nixal_reprap4040_XtensionerHolder (Autodesk Fusion 360 design; units mm, degrees)
Autodesk Fusion 360 part; units mm, degrees
sketch "Sketch1" plane through (0, 0, 0) normal (0, 1, 0) x (1, 0, 0)
  line L0 (2, 0) -> (6.3, 0)
  line L1 (8.3, 2) -> (8.3, 22.7)
  line L2 (6.3, 24.7) -> (2, 24.7)
  line L3 (0, 22.7) -> (0, 2)
  line L4 (-2, 26.2) -> (10.3, 26.2)
  line L5 (12.3, 24.2) -> (12.3, 0.5)
  line L6 (10.3, -1.5) -> (-2, -1.5)
  line L7 (-4, 0.5) -> (-4, 24.2)
  line L8 (0, 24.7) -> (8.3, 0) construction
  line L9 (8.3, 24.7) -> (0, 0) construction
  circle A0 centre (4.15, 12.35) radius 1.65
  line L10 (7.4, 9.1) -> (0.9, 15.6) construction
  line L11 (0.9, 9.1) -> (7.4, 15.6) construction
  circle A1 centre (4.15, 12.35) radius 3.25
  arc A2 (2, 24.7) -> (0, 22.7) centre (2, 22.7) ccw
  arc A3 (8.3, 22.7) -> (6.3, 24.7) centre (6.3, 22.7) ccw
  arc A4 (0, 2) -> (2, 0) centre (2, 2) ccw
  arc A5 (6.3, 0) -> (8.3, 2) centre (6.3, 2) ccw
  arc A6 (-2, 26.2) -> (-4, 24.2) centre (-2, 24.2) ccw
  arc A7 (12.3, 24.2) -> (10.3, 26.2) centre (10.3, 24.2) ccw
  arc A8 (-4, 0.5) -> (-2, -1.5) centre (-2, 0.5) ccw
  arc A9 (10.3, -1.5) -> (12.3, 0.5) centre (10.3, 0.5) ccw
  dimension "d1" = 24.7
  dimension "d2" = 8.3
  dimension "d3" = 4
  dimension "d4" = 4
  dimension "d5" = 1.5
  dimension "d6" = 1.5
  dimension "d7" = 3.3
  dimension "d15" = 6.5
  dimension "d18" = 2
  dimension "d19" = 2
  dimension "d20" = 2
  dimension "d21" = 2
  dimension "d22" = 2
  dimension "d23" = 2
  dimension "d24" = 2
  dimension "d25" = 2
  constraint horizontal L0
  constraint vertical L1
  constraint horizontal L2
  constraint vertical L3
  constraint horizontal L4
  constraint vertical L5
  constraint horizontal L6
  constraint vertical L7
  constraint coincident L9.end origin
  constraint midpoint L9
  constraint coincident L10
  constraint coincident L11
  constraint tangent L2 A2
  constraint tangent L3 A2
  constraint tangent L2 A3
  constraint tangent L1 A3
  constraint tangent L3 A4
  constraint tangent L0 A4
  constraint tangent L1 A5
  constraint tangent L0 A5
  constraint tangent L4 A6
  constraint tangent L7 A6
  constraint tangent L4 A7
  constraint tangent L5 A7
  constraint tangent L7 A8
  constraint tangent L6 A8
  constraint tangent L5 A9
  constraint tangent L6 A9
  measures "d1" distance of L9.end
  measures "d3" distance of L1 L5
  measures "d4" distance of L3 L7
  measures "d5" distance of L2 L4
  measures "d6" distance of L0 L6
  measures "d7" diameter of A0
  measures "d15" diameter of A1
  measures "d18" radius of A2
  measures "d19" radius of A3
  measures "d20" radius of A4
  measures "d21" radius of A5
  measures "d22" radius of A6
  measures "d23" radius of A7
  measures "d24" radius of A8
  measures "d25" radius of A9
extrude "Extrude1" add sketch "Sketch1" along normal blind 3 contours L0 L1 L2 L3 A2 A3 A4 A5 | L4 L5 L6 L7 A6 A7 A8 A9 | A1 makes body 1
extrude "Extrude2" add sketch "Sketch1" along normal blind 10 and the other way blind -3 separate body contours L0 L1 L2 L3 A2 A3 A4 A5 | A1 makes body 2
extrude "Extrude3" cut sketch "Sketch1" along normal blind 6 contours A1 bodies 1 2
